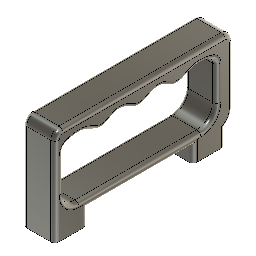
main_handle (Autodesk Fusion 360 design; units mm, degrees)
Autodesk Fusion 360 part; units mm, degrees
sketch "Skizze1" plane through (0, 0, 0) normal (1, 0, 0) x (0, 1, 0)
  line L0 (0, 0) -> (0, 60)
  line L1 (0, 60) -> (111.25, 60)
  line L2 (111.25, 60) -> (111.25, 10)
  line L3 (111.25, 10) -> (106.25, 10)
  line L4 (106.25, 10) -> (106.25, 0)
  line L5 (106.25, 0) -> (86.25, 0)
  line L6 (86.25, 0) -> (86.25, 10)
  line L7 (86.25, 10) -> (20, 10)
  line L8 (20, 10) -> (20, 0)
  line L9 (20, 0) -> (0, 0)
  dimension "d1" = 20
  dimension "d2" = 20
  dimension "d3" = 86.25
  dimension "d4" = 5
  dimension "d5" = 60
  dimension "d6" = 10
  dimension "d7" = 10
  constraint coincident L0.start L9.end
  constraint vertical L0
  constraint perpendicular L0 L1
  constraint perpendicular L1 L2
  constraint perpendicular L2 L3
  constraint perpendicular L3 L4
  constraint perpendicular L4 L5
  constraint perpendicular L3 L6
  constraint perpendicular L6 L7
  constraint perpendicular L3 L8
  constraint perpendicular L0 L9
  constraint collinear L5 L9
  measures "d1" distance of L8.end L0.start
  measures "d2" distance of L4.end L5.end
  measures "d3" distance of L0 L6
  measures "d4" distance of L2.end L3.end
  measures "d5" distance of L0.start L0.end
  measures "d6" distance of L7.end L8.end
  measures "d7" distance of L3.end L4.end
extrude "Extrusion1" add sketch "Skizze1" along normal mid plane 20
sketch "Skizze2" plane through (10, 0, 0) normal (1, 0, 0) x (0, 1, 0)
  line L0 (20, 0) -> (20, 10)
  line L1 (20, 10) -> (86.25, 10)
  line L2 (86.25, 10) -> (86.25, 0)
  line L3 (86.25, 0) -> (106.25, 0)
  line L4 (106.25, 0) -> (106.25, 10)
  line L5 (106.25, 10) -> (111.25, 10)
  line L6 (111.25, 10) -> (111.25, 60)
  line L7 (111.25, 60) -> (0, 60)
  line L8 (0, 60) -> (0, 0)
  line L9 (0, 0) -> (20, 0)
  spline S0 degree 5 poles (5, 50) (5.4629, 50.1553) (6.3735, 50.4513) (7.694, 50.8519) (9.3638, 51.2991) (11.3005, 51.7132) (13.0897, 51.9831) (14.7376, 52.1102) (16.2549, 52.0972) (17.6578, 51.9482) (18.9696, 51.669) (20.2192, 51.2688) (21.4368, 50.7637) (22.6495, 50.1803) (23.8773, 49.5586) (25.128, 48.9571) (26.3991, 48.445) (27.6823, 48.0889) (28.9673, 47.9419) (30.2456, 48.0313) (31.5144, 48.3467) (32.7751, 48.8486) (34.0317, 49.4766) (35.2885, 50.1586) (36.5487, 50.8196) (37.8129, 51.3893) (39.0803, 51.8072) (40.349, 52.0283) (41.6173, 52.0271) (42.8839, 51.8047) (44.1488, 51.3883) (45.4125, 50.8244) (46.6756, 50.1733) (47.9391, 49.5031) (49.2032, 48.8845) (50.4682, 48.3839) (51.7339, 48.0572) (53, 47.9433) (54.2661, 48.0572) (55.5318, 48.3839) (56.7968, 48.8845) (58.0609, 49.5031) (59.3244, 50.1733) (60.5875, 50.8244) (61.8512, 51.3883) (63.1161, 51.8047) (64.3827, 52.0271) (65.651, 52.0283) (66.9197, 51.8072) (68.1871, 51.3893) (69.4513, 50.8196) (70.7115, 50.1586) (71.9683, 49.4766) (73.2249, 48.8486) (74.4856, 48.3467) (75.7544, 48.0313) (77.0327, 47.9419) (78.3177, 48.0889) (79.6009, 48.445) (80.872, 48.9571) (82.1227, 49.5586) (83.3505, 50.1803) (84.5632, 50.7637) (85.7808, 51.2688) (87.0304, 51.669) (88.3422, 51.9482) (89.7451, 52.0972) (91.2624, 52.1102) (92.9103, 51.9831) (94.6995, 51.7132) (96.6362, 51.2991) (98.306, 50.8519) (99.6265, 50.4513) (100.5371, 50.1553) (101, 50) knots 0 0 0 0 0 0 0.01428571 0.02857143 0.04285714 0.05714286 0.07142857 0.08571429 0.1 0.11428571 0.12857143 0.14285714 0.15714286 0.17142857 0.18571429 0.2 0.21428571 0.22857143 0.24285714 0.25714286 0.27142857 0.28571429 0.3 0.31428571 0.32857143 0.34285714 0.35714286 0.37142857 0.38571429 0.4 0.41428571 0.42857143 0.44285714 0.45714286 0.47142857 0.48571429 0.5 0.51428571 0.52857143 0.54285714 0.55714286 0.57142857 0.58571429 0.6 0.61428571 0.62857143 0.64285714 0.65714286 0.67142857 0.68571429 0.7 0.71428571 0.72857143 0.74285714 0.75714286 0.77142857 0.78571429 0.8 0.81428571 0.82857143 0.84285714 0.85714286 0.87142857 0.88571429 0.9 0.91428571 0.92857143 0.94285714 0.95714286 0.97142857 0.98571429 1 1 1 1 1 1
  line L10 (5, 50) -> (101, 50)
  line L11 (5, 50) -> (5, 15)
  line L12 (5, 15) -> (101, 15)
  line L13 (101, 15) -> (101, 50)
  point P0 (17, 52)
  point P1 (23, 50)
  point P2 (29, 48)
  point P3 (35, 50)
  point P4 (41, 52)
  point P5 (47, 50)
  point P6 (53, 48)
  point P7 (59, 50)
  point P8 (65, 52)
  point P9 (71, 50)
  point P10 (77, 48)
  point P11 (83, 50)
  point P12 (89, 52)
  dimension "d10" = 5
  dimension "d11" = 12
  dimension "d12" = 6
  dimension "d13" = 6
  dimension "d14" = 6
  dimension "d15" = 6
  dimension "d16" = 6
  dimension "d17" = 6
  dimension "d18" = 6
  dimension "d19" = 6
  dimension "d20" = 6
  dimension "d21" = 6
  dimension "d22" = 6
  dimension "d24" = 10
  dimension "d25" = 10
  dimension "d26" = 6
  dimension "d27" = 12
  dimension "d28" = 2
  dimension "d29" = 2
  dimension "d30" = 2
  dimension "d31" = 2
  dimension "d32" = 2
  dimension "d33" = 2
  dimension "d34" = 2
  dimension "d35" = 35
  constraint coincident P1 L10
  constraint coincident P3 L10
  constraint coincident P5 L10
  constraint coincident P7 L10
  constraint coincident P9 L10
  constraint coincident P11 L10
  constraint perpendicular L10 L11
  constraint perpendicular L11 L12
  constraint perpendicular L10 L13
  measures "d10" distance of L8 S0.start
  measures "d11" distance of S0.start P0
  measures "d12" horizontal distance of P0 P1
  measures "d13" horizontal distance of P1 P2
  measures "d14" horizontal distance of P2 P3
  measures "d15" horizontal distance of P3 P4
  measures "d16" horizontal distance of P4 P5
  measures "d17" horizontal distance of P5 P6
  measures "d18" horizontal distance of P6 P7
  measures "d19" horizontal distance of P7 P8
  measures "d20" horizontal distance of P8 P9
  measures "d21" horizontal distance of P9 P10
  measures "d22" horizontal distance of P10 P11
  measures "d24" distance of L7 S0.end
  measures "d25" distance of L7 S0.start
  measures "d26" horizontal distance of P11 P12
  measures "d27" distance of S0.end P12
  measures "d28" distance of L10 P12
  measures "d29" distance of P10 L10
  measures "d30" distance of P8 L10
  measures "d31" distance of P6 L10
  measures "d32" distance of P4 L10
  measures "d33" distance of P2 L10
  measures "d34" distance of P0 L10
  measures "d35" distance of S0.start L11.end
extrude "Extrusion2" cut sketch "Skizze2" against normal through all contours S0 L10 | S0 L10 L11 L12 L13 | S0 L10 | S0 L10 | S0 L10 picked at (13.1167, 50.5643) picked at (39.3753, 50.6892) picked at (93.7853, 50.364) picked at (66.4503, 50.2815)
fillet "Abrundung11" radius 10 3 edges at (0, 101, 15) (0, 111.25, 10) (0, 5, 15)
fillet "Abrundung12" radius 5 2 edges at (0, 111.25, 60) (0, 0, 60)
fillet "Abrundung13" radius 5 2 edges at (0, 101, 50) (0, 5, 50)
fillet "Abrundung14" radius 2.5 28 edges at (-10, 0, 27.5) (-10, 1.4645, 58.5355) (-10, 55.625, 60) (-10, 109.7855, 58.5355) (-10, 111.25, 36.8301) (-10, 109.9103, 13.6603) (-10, 6.0478, 49.3407) (-10, 53, 48) (-10, 99.9489, 49.3449) (-10, 101, 35.639) (-10, 98.0711, 17.9289) (-10, 53, 15) (-10, 7.9289, 17.9289) (-10, 5, 35.639) (10, 7.9289, 17.9289) (10, 53, 15) (10, 98.0711, 17.9289) (10, 101, 35.639) (10, 99.9522, 49.3407) (10, 53, 48) (10, 6.0511, 49.3449) (10, 5, 35.639) (10, 109.9103, 13.6603) (10, 111.25, 36.8301) (10, 109.7855, 58.5355) (10, 55.625, 60) (10, 1.4645, 58.5355) (10, 0, 27.5)
fillet "Abrundung15" radius 2.5 2 edges at (-10, 53.125, 10) (10, 53.125, 10)
fillet "Abrundung16" radius 2.5 6 edges at (-10, 86.25, 6.25) (10, 86.25, 6.25) (10, 106.25, 6.535) (-10, 106.25, 6.535) (-10, 20, 6.25) (10, 20, 6.25)
sketch "Skizze3" plane through (0, 0, 0) normal (0, 0, -1) x (1, 0, 0)
  arc A0 (-10, -103.75) -> (-7.5, -106.25) centre (-7.5, -103.75) ccw
  line L0 (-7.5, -106.25) -> (7.5, -106.25)
  arc A1 (7.5, -106.25) -> (10, -103.75) centre (7.5, -103.75) ccw
  line L1 (10, -103.75) -> (10, -88.75)
  arc A2 (10, -88.75) -> (7.5, -86.25) centre (7.5, -88.75) ccw
  line L2 (7.5, -86.25) -> (-7.5, -86.25)
  arc A3 (-7.5, -86.25) -> (-10, -88.75) centre (-7.5, -88.75) ccw
  line L3 (-10, -88.75) -> (-10, -103.75)
  line L4 (0, -1.75) -> (0, -22.5)
  point P0 (0, -96.25)
  point P1 (0, -10)
  dimension "d69" = 86.25
  dimension "d70" = 10
  constraint coincident P1 L4
  constraint coincident P0 L4
  measures "d69" distance of P0 P1
  measures "d70" distance of L0 P0
hole "Bohrung1" at (0, 96.25, 0) at (0, 10, 0) direction (0, 0, 1) diameter 3.2 depth 14 tip angle 180
ref_plane "Arbeitsebene2" through (0, 96.25, 5) normal (0, 0, -1) x (0, 1, 0)
sketch "Skizze12" plane through (0, 96.25, 5) normal (0, 0, -1) x (1, 0, 0)
  line L0 (2.9, 89.85) -> (-2.9, 89.85)
  line L1 (-2.9, 89.85) -> (-2.9, -3.6)
  line L2 (-2.9, -3.6) -> (2.9, -3.6)
  line L3 (2.9, -3.6) -> (2.9, 89.85)
  point P0 (-1.6, 86.25)
  dimension "d119" = 5.8
  dimension "d120" = 3.6
  dimension "d121" = 2.9
  dimension "d122" = 3.6
  constraint horizontal L0
  constraint vertical L1
  constraint horizontal L2
  constraint vertical L3
  measures "d119" distance of L1.end L2.end
  measures "d120" distance of origin L2
  measures "d121" distance of origin L3
  measures "d122" vertical distance of L0.end P0
extrude "Extrusion10" cut sketch "Skizze12" against normal blind 3
sketch "Skizze13" plane through (0, 0, 0) normal (1, 0, 0) x (0, 1, 0)
  line L0 (111.25, 18.6603) -> (111.25, 55)
  line L1 (88.75, 0) -> (103.75, 0)
  line L2 (111.25, 50) -> (106.75, 50)
  line L3 (106.75, 50) -> (106.75, 45)
  line L4 (106.75, 45) -> (104.75, 45)
  line L5 (104.75, 45) -> (104.75, 19.017)
  line L6 (104.75, 19.017) -> (102.25, 15.4466)
  line L7 (102.25, 15.4466) -> (102.25, 0)
  line L8 (105.25, 0) -> (105.25, 14.5007)
  line L9 (105.25, 14.5007) -> (107, 17)
  line L10 (107, 17) -> (107, 42.5)
  line L11 (107, 42.5) -> (108.25, 42.5)
  line L12 (108.25, 42.5) -> (108.25, 43.5)
  line L13 (108.25, 43.5) -> (111.25, 43.5)
  line L14 (111.25, 43.5) -> (111.25, 50)
  line L15 (106.25, 60) -> (5, 60)
  line L16 (102.25, 0) -> (105.25, 0)
  dimension "d128" = 4.5
  dimension "d129" = 2
  dimension "d130" = 3
  dimension "d131" = 2.25
  dimension "d132" = 2.5
  dimension "d133" = 5
  dimension "d134" = 6.5
  dimension "d135" = 10
  dimension "d137" = 145
  dimension "d138" = 2.5
  dimension "d139" = 3
  dimension "d140" = 3
  dimension "d141" = 28
  constraint coincident L0 L2.start
  constraint perpendicular L0 L2
  constraint perpendicular L2 L3
  constraint perpendicular L3 L4
  constraint perpendicular L4 L5
  constraint coincident L1 L7.end
  constraint perpendicular L1 L7
  constraint coincident L1 L8.start
  constraint perpendicular L1 L8
  constraint parallel L6 L9
  constraint perpendicular L1 L10
  constraint perpendicular L7 L11
  constraint perpendicular L11 L12
  constraint coincident L0 L13.end
  constraint perpendicular L0 L13
  measures "d128" distance of L2.start L2.end
  measures "d129" distance of L3.end L4.end
  measures "d130" distance of L12.end L13.end
  measures "d131" distance of L5 L10
  measures "d132" distance of L4 L11
  measures "d133" distance of L2.end L3.end
  measures "d134" distance of L2.start L13.end
  measures "d135" distance of L2 L15
  measures "d137" angle of L5 L6
  measures "d138" horizontal distance of L5.end L6.end
  measures "d139" distance of L7 L8
  measures "d140" distance of L6 L9
  measures "d141" vertical distance of L4.end L9.end
extrude "Extrusion11" cut sketch "Skizze13" along normal mid plane 6.5
equation "d11 = fingerdist * 2"
equation "d12 = fingerdist"
equation "d13 = fingerdist"
equation "d14 = fingerdist"
equation "d15 = fingerdist"
equation "d16 = fingerdist"
equation "d17 = fingerdist"
equation "d18 = fingerdist"
equation "d19 = fingerdist"
equation "d20 = fingerdist"
equation "d21 = fingerdist"
equation "d22 = fingerdist"
equation "d26 = fingerdist"
equation "d27 = fingerdist * 2"
equation "fingerdist = 6 mm"
